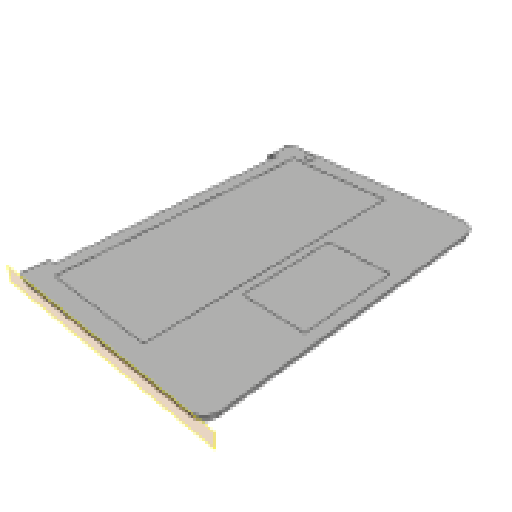
# Autodesk Inventor part: dellLatitudeBase
Saved by Autodesk Inventor 2025 (Build 290162000, 162)
## iProperties
Created: 2024-12-07
Part Number: dellLatitudeBase
Material: Generic
Document SubType Name: Modeling
Designer: derm
Density: 1 g/cm^3
Appearance: Smooth - Medium Gray
Author: derm
Autodesk Inventor part; units mm, degrees
ref_plane "YZ Plane" through (0, 0, 0) normal (1, 0, 0) x (0, 1, 0)
ref_plane "XZ Plane" through (0, 0, 0) normal (0, 1, 0) x (-1, 0, 0)
sketch "Sketch1" plane through (0, 0, 0) normal (0, 1, 0) x (-1, 0, 0)
  line L0 (-101.6, 165.1) -> (101.6, 165.1)
  line L1 (117.475, 149.225) -> (117.475, -149.225)
  line L2 (101.6, -165.1) -> (-101.6, -165.1)
  line L3 (-117.475, -149.225) -> (-117.475, 149.225)
  line L4 (-117.475, 165.1) -> (117.475, -165.1) construction
  line L5 (117.475, 165.1) -> (-117.475, -165.1) construction
  arc A0 (-101.6, 165.1) -> (-117.475, 149.225) centre (-101.6, 149.225) ccw
  arc A1 (-117.475, -149.225) -> (-101.6, -165.1) centre (-101.6, -149.225) ccw
  arc A2 (101.6, -165.1) -> (117.475, -149.225) centre (101.6, -149.225) ccw
  arc A3 (117.475, 149.225) -> (101.6, 165.1) centre (101.6, 149.225) ccw
  point P0 (0, 0)
  dimension "d0" = 330.2
  dimension "d1" = 234.95
  dimension "d2" = 15.875
  constraints: 12 end point, 8 point on circle, 8 point on line, 8 tangent, 4 centre point, 3 equal radius, 2 midpoint, 2 parallel, 1 horizontal, 1 perpendicular
  measures "d0" distance of L5.start L4.end
  measures "d1" distance between parallel lines of L3 L1
  measures "d2" radius of A0
extrude "Extrusion1" add sketch "Sketch1" against normal blind 15.3035
sketch "Sketch2" plane through (0, 0, 0) normal (0, 1, 0) x (1, 0, 0)
  line L0 (101.6, 165.1) -> (-101.6, 165.1) projected
  arc A0 (-101.6, 165.1) -> (-117.475, 149.225) centre (-101.6, 149.225) ccw projected
  line L1 (-117.475, 149.225) -> (-117.475, -149.225) projected
  arc A1 (-117.475, -149.225) -> (-101.6, -165.1) centre (-101.6, -149.225) ccw projected
  line L2 (-101.6, -165.1) -> (101.6, -165.1) projected
  arc A2 (101.6, -165.1) -> (117.475, -149.225) centre (101.6, -149.225) ccw projected
  line L3 (117.475, -149.225) -> (117.475, 149.225) projected
  arc A3 (117.475, 149.225) -> (101.6, 165.1) centre (101.6, 149.225) ccw projected
  line L4 (28.8925, -144.4625) -> (-88.265, -144.4625)
  line L5 (-88.265, -144.4625) -> (-88.265, 144.4625)
  line L6 (-88.265, 144.4625) -> (28.8925, 144.4625)
  line L7 (28.8925, 144.4625) -> (28.8925, -144.4625)
  line L8 (28.8925, -144.4625) -> (-88.265, 144.4625) construction
  line L9 (-88.265, -144.4625) -> (28.8925, 144.4625) construction
  line L10 (104.4575, -52.3875) -> (38.4175, -52.3875)
  line L11 (38.4175, -52.3875) -> (38.4175, 52.3875)
  line L12 (38.4175, 52.3875) -> (104.4575, 52.3875)
  line L13 (104.4575, 52.3875) -> (104.4575, -52.3875)
  line L14 (104.4575, -52.3875) -> (38.4175, 52.3875) construction
  line L15 (38.4175, -52.3875) -> (104.4575, 52.3875) construction
  circle A4 centre (-76.6206, 156.377) radius 5.1319
  point P0 (0, 0)
  point P1 (-29.6863, 0)
  point P2 (71.4375, 0)
  point P3 (71.4375, 52.3875)
  dimension "d5" = 20.6375
  dimension "d6" = 20.6375
  dimension "d7" = 29.21
  dimension "d8" = 117.1575
  dimension "d9" = 104.775
  dimension "d10" = 66.04
  dimension "d11" = 9.525
  constraints: 24 end point, 5 midpoint, 4 parallel, 2 horizontal, 2 perpendicular, 1 centre point
  measures "d5" distance between parallel lines of L0 L6
  measures "d6" distance between parallel lines of L2 L4
  measures "d7" distance between parallel lines of L1 L5
  measures "d8" distance between parallel lines of L5 L7
  measures "d9" distance from line of point (71.437, 52.387) L10
  measures "d10" distance between parallel lines of L11 L13
  measures "d11" distance between parallel lines of L7 L11
extrude "Extrusion2" cut sketch "Sketch2" against normal blind 0.254 contours L4 L5 L6 L7 | L10 L11 L12 L13 | A4
fillet "Fillet1" radius 15.875 8 edges at (-117.475, -15.3035, 0) (-112.8253, -15.3035, -160.4503) (0, -15.3035, -165.1) (112.8253, -15.3035, -160.4503) (117.475, -15.3035, 0) (112.8253, -15.3035, 160.4503) (0, -15.3035, 165.1) (-112.8253, -15.3035, 160.4503)
sketch "Sketch3" plane through (0, 0, 0) normal (0, 1, 0) x (1, 0, 0)
  circle A0 centre (-76.6206, 156.377) radius 5.1319 projected
  line L0 (38.4175, -52.3875) -> (38.4175, 52.3875) projected
  line L1 (38.4175, 52.3875) -> (104.4575, 52.3875) projected
  line L2 (104.4575, 52.3875) -> (104.4575, -52.3875) projected
  line L3 (104.4575, -52.3875) -> (38.4175, -52.3875) projected
  line L4 (-88.265, -144.4625) -> (-88.265, 144.4625) projected
  line L5 (-88.265, 144.4625) -> (28.8925, 144.4625) projected
  line L6 (28.8925, 144.4625) -> (28.8925, -144.4625) projected
  line L7 (28.8925, -144.4625) -> (-88.265, -144.4625) projected
  line L8 (101.6, 165.1) -> (-101.6, 165.1) projected
  arc A1 (-101.6, 165.1) -> (-117.475, 149.225) centre (-101.6, 149.225) ccw projected
  line L9 (-117.475, 149.225) -> (-117.475, -149.225) projected
  arc A2 (-117.475, -149.225) -> (-101.6, -165.1) centre (-101.6, -149.225) ccw projected
  line L10 (-101.6, -165.1) -> (101.6, -165.1) projected
  arc A3 (101.6, -165.1) -> (117.475, -149.225) centre (101.6, -149.225) ccw projected
  line L11 (117.475, -149.225) -> (117.475, 149.225) projected
  arc A4 (117.475, 149.225) -> (101.6, 165.1) centre (101.6, 149.225) ccw projected
  line L12 (-117.475, -166.6875) -> (117.475, -166.6875)
  line L13 (117.475, -166.6875) -> (117.475, 166.6875)
  line L14 (117.475, 166.6875) -> (-117.475, 166.6875)
  line L15 (-117.475, 166.6875) -> (-117.475, -166.6875)
  line L16 (-117.475, 166.6875) -> (-103.505, 166.6875)
  line L17 (-103.505, 166.6875) -> (-103.505, 134.9375)
  line L18 (-103.505, 134.9375) -> (-117.475, 134.9375)
  line L19 (-117.475, 134.9375) -> (-117.475, 166.6875)
  line L20 (-117.475, -166.6875) -> (-103.505, -166.6875)
  line L21 (-103.505, -166.6875) -> (-103.505, -134.9375)
  line L22 (-103.505, -134.9375) -> (-117.475, -134.9375)
  line L23 (-117.475, -134.9375) -> (-117.475, -166.6875)
  line L24 (-103.505, -134.9375) -> (-117.475, -134.9375)
  line L25 (-117.475, -134.9375) -> (-117.475, 134.9375)
  line L26 (-117.475, 134.9375) -> (-103.505, 134.9375)
  line L27 (-103.505, 134.9375) -> (-103.505, -134.9375)
  point P0 (0, 0)
  point P1 (-110.49, 166.6875)
  point P2 (-110.49, 134.9375)
  point P3 (-110.49, -134.9375)
  dimension "d15" = 31.75
  dimension "d16" = 31.75
  dimension "d17" = 13.97
  constraints: 32 end point, 8 parallel, 4 horizontal, 4 perpendicular, 3 midpoint, 1 point on line, 2 other
  measures "d15" distance of point (-110.49, 166.688) point (-110.49, 134.938)
  measures "d16" distance from line of point (-110.49, -134.938) L12
  measures "d17" distance between parallel lines of L25 L27
extrude "Extrusion3" cut sketch "Sketch3" against normal through all contours L27 L22 L9 L18
sketch "Sketch4" plane through (0, 0, 0) normal (0, 0, 1) x (1, 0, 0)
  arc A0 (-117.475, 0) -> (-103.505, -15.19) centre (-101.6103, 0.5715) ccw projected
  line L0 (-103.505, 0) -> (-117.475, 0) projected
  line L1 (-103.505, 0) -> (-103.505, -15.19) projected
  circle A1 centre (-109.8636, -6.6929) radius 3.8393
  point P0 (0, 0)
  constraints: 1 centre point
extrude "Extrusion4" cut sketch "Sketch4" along normal mid plane 300 contours A1
sketch "Sketch5" plane through (-117.475, 0, -134.9375) normal (0, 0, 1) x (1, 0, 0)
  circle A0 centre (7.6114, -6.6929) radius 3.8393 projected
  arc A1 (0, 0) -> (13.97, -15.19) centre (15.8647, 0.5715) ccw projected
  line L0 (13.97, 0) -> (13.97, -15.19) projected
  line L1 (0, 0) -> (13.97, 0) projected
  arc A2 (6.7579, 0) -> (2.4095, -7.853) centre (6.7579, -5.1304) ccw
  arc A3 (0, 0) -> (13.97, -15.19) centre (15.8647, 0.5715) ccw projected
  line L2 (0, 0) -> (13.97, 0) projected
  point P0 (117.475, 0)
  point P1 (2.4095, -7.853)
  point P2 (6.7579, 0)
  constraints: 3 point on circle, 3 tangent, 1 centre point, 1 point on line
extrude "Extrusion5" cut sketch "Sketch5" along normal through all both and the other way through all contours L1 A2 A1
ref_plane "Work Plane2" through (-101.6, 0, 165.1) normal (0, 0, 1) x (1, 0, 0)
sketch "Sketch6" plane through (-101.6, 0, 165.1) normal (0, 0, 1) x (1, 0, 0)
  arc A0 (-13.4655, -7.853) -> (-0.0103, -15.3035) centre (-0.0103, 0.5715) ccw projected
  line L0 (-0.0103, -15.3035) -> (0, -15.3035) projected
  line L1 (0, -15.3035) -> (0, 0) projected
  line L2 (-9.1171, 0) -> (0, 0) projected
  line L3 (203.2, -15.3035) -> (203.2, 0) projected
  line L4 (0, 0) -> (203.2, 0) projected
  line L5 (0, -15.3035) -> (0, 0) projected
  line L6 (0, -15.3035) -> (203.2, -15.3035) projected
  circle A1 centre (0, -7.6518) radius 3.2401
  line L7 (10.3708, -10.7389) -> (25.3478, -10.7389)
  line L8 (25.3478, -10.7389) -> (25.3478, -4.5646)
  line L9 (25.3478, -4.5646) -> (10.3708, -4.5646)
  line L10 (10.3708, -4.5646) -> (10.3708, -10.7389)
  line L11 (10.3708, -10.7389) -> (25.3478, -4.5646) construction
  line L12 (25.3478, -10.7389) -> (10.3708, -4.5646) construction
  line L13 (88.2734, -10.7389) -> (105.1829, -10.7389)
  line L14 (105.1829, -10.7389) -> (105.1829, -4.5646)
  line L15 (105.1829, -4.5646) -> (88.2734, -4.5646)
  line L16 (88.2734, -4.5646) -> (88.2734, -10.7389)
  line L17 (88.2734, -10.7389) -> (105.1829, -4.5646) construction
  line L18 (105.1829, -10.7389) -> (88.2734, -4.5646) construction
  arc A2 (-9.1171, 0) -> (-13.4655, -7.853) centre (-9.1171, -5.1304) ccw projected
  line L19 (36.8221, -10.6503) -> (56.8718, -10.6503)
  line L20 (56.8718, -10.6503) -> (56.8718, -4.6532)
  line L21 (56.8718, -4.6532) -> (36.8221, -4.6532)
  line L22 (36.8221, -4.6532) -> (36.8221, -10.6503)
  line L23 (36.8221, -10.6503) -> (56.8718, -4.6532) construction
  line L24 (56.8718, -10.6503) -> (36.8221, -4.6532) construction
  point P0 (101.6, 0)
  point P1 (17.8593, -7.6518)
  point P2 (96.7281, -7.6518)
  point P3 (105.1829, -7.6517)
  point P4 (46.8469, -7.6517)
  dimension "d24" = 114.3
  constraints: 36 end point, 8 midpoint, 6 parallel, 3 horizontal, 3 perpendicular, 1 centre point, 2 other
  measures "d24" horizontal distance of point (105.183, -7.652) A2.centre
extrude "Extrusion6" cut sketch "Sketch6" against normal blind 10 contours A1 L1 | L1 A1 | L10 L9 L8 L7 | L16 L15 L14 L13 | L22 L21 L20 L19
mirror "Mirror2" about plane through (0, 0, 0) normal (0, 0, 1) of "Extrusion6"
body "Solid1"
